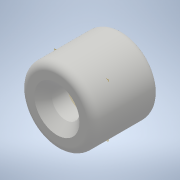
# Autodesk Inventor part: ПодпорныйКаток
Saved by Autodesk Inventor 2020 (Build 240168000, 168)
## iProperties
Created: 2021-05-10
Part Number: ПодпорныйКаток
Material: Типовые
Document SubType Name: Modeling
Designer: I_Love_U_Bogdan
Density: 1 g/cm^3
Appearance: По умолчанию
Author: I_Love_U_Bogdan
Autodesk Inventor part; units mm, degrees
ref_plane "YZ Plane" through (0, 0, 0) normal (1, 0, 0) x (0, 1, 0)
ref_plane "XZ Plane" through (0, 0, 0) normal (0, 1, 0) x (-1, 0, 0)
ref_plane "XY Plane" through (0, 0, 0) normal (0, 0, 1) x (1, 0, 0)
sketch "Эскиз1" plane through (0, 0, 0) normal (0, 0, 1) x (1, 0, 0)
  circle A0 centre (0, 0) radius 6.6
  circle A1 centre (0, 0) radius 10.6
  dimension "d0" = 13.2
  dimension "d1" = 4
  constraints: 2 centre point, 2 coincident
  measures "d0" diameter of A0
  measures "d1" radial gap between concentric circles of A0 A1
extrude "Выдавливание1" add sketch "Эскиз1" along normal blind 7 and the other way blind 12
fillet "Сопряжение1" radius 2 2 edges at (-10.6, 0, 7) (-10.6, 0, -12)
chamfer "Фаска1" distance 1 angle 45 1 edges at (-6.6, 0, -12)
ref_plane "РабПлоскость1" through (0, 0, 0) normal (0, 0, 1) x (1, 0, 0)
sketch "Эскиз2" plane through (0, 0, 0) normal (0, 0, 1) x (1, 0, 0)
  circle A0 centre (0, 0) radius 4
  circle A1 centre (0, 0) radius 8.6 projected
  circle A2 centre (0, 0) radius 7.5
  dimension "d10" = 8
  dimension "d11" = 15
  constraints: 2 centre point, 2 coincident
  measures "d10" diameter of A0
  measures "d11" diameter of A2
extrude "Выдавливание2" add sketch "Эскиз2" along normal blind 7 contours A2
chamfer "Фаска2" distance 2.5 angle 45 1 edges at (-4, 0, 7)
